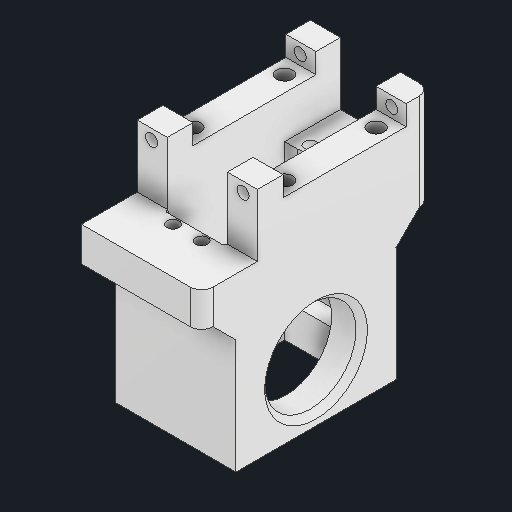
# Autodesk Inventor part: VerticalAxisServoMount
Saved by Autodesk Inventor 2025 (Build 290162000, 162)
## iProperties
Created: 2024-01-29
Part Number: VerticalAxisServoMount
Material: PC/ABS Plastic
Document SubType Name: Modeling
Designer: avsar
Density: 1.1 g/cm^3
Appearance: Smooth - White
Author: avsar
Autodesk Inventor part; units mm, degrees
ref_plane "YZ Plane" through (0, 0, 0) normal (1, 0, 0) x (0, 1, 0)
ref_plane "XZ Plane" through (0, 0, 0) normal (0, 1, 0) x (-1, 0, 0)
ref_plane "XY Plane" through (0, 0, 0) normal (0, 0, 1) x (1, 0, 0)
sketch "Sketch1" plane through (0, 0, 0) normal (1, 0, 0) x (0, 1, 0)
  circle A0 centre (0, 0) radius 15.95
  dimension "d0" = 31.9
  constraints: 1 centre point, 1 coincident
  measures "d0" diameter of A0
extrude "Extrusion1" add sketch "Sketch1" along normal blind 8
sketch "Sketch2" plane through (8, 0, 0) normal (1, 0, 0) x (0, 0, -1)
  line L0 (-28, -20) -> (28, -20)
  line L1 (28, -20) -> (28, 40)
  line L2 (28, 40) -> (-28, 40)
  line L3 (-28, 40) -> (-28, -20)
  line L4 (-28, -20) -> (28, 40) construction
  line L5 (28, -20) -> (-28, 40) construction
  point P0 (0, 0)
  point P1 (0, 10)
  point P2 (0, 10)
  dimension "d3" = 60
  dimension "d4" = 56
  dimension "d46" = 10
  constraints: 12 end point, 2 midpoint, 2 parallel, 1 horizontal, 1 perpendicular, 1 vertical alignment
  measures "d3" distance of L1.end L0.end
  measures "d4" distance of L1.end L2.end
  measures "d46" distance of point (0, 0) point (0, 10)
extrude "Extrusion2" add sketch "Sketch2" along normal blind 42
sketch "Sketch3" plane through (8, 40, 28) normal (0, 1, 0) x (1, 0, 0)
  line L0 (0, 56) -> (42, 56) projected
  line L1 (21, 56) -> (21, 0) construction
  line L2 (0, 0) -> (42, 0) projected
  line L3 (10.5, 7.5) -> (31.5, 7.5)
  line L4 (31.5, 7.5) -> (31.5, 48.5)
  line L5 (31.5, 48.5) -> (10.5, 48.5)
  line L6 (10.5, 48.5) -> (10.5, 7.5)
  line L7 (10.5, 7.5) -> (31.5, 48.5) construction
  line L8 (31.5, 7.5) -> (10.5, 48.5) construction
  point P0 (-8, 28)
  point P1 (21, 28)
  dimension "d7" = 21
  dimension "d8" = 41
  constraints: 14 end point, 5 midpoint, 2 parallel, 1 horizontal, 1 perpendicular
  measures "d7" distance of L5.end L4.end
  measures "d8" distance of L4.end L3.end
extrude "Extrusion3" cut sketch "Sketch3" against normal through all
sketch "Sketch4" plane through (50, 0, 0) normal (1, 0, 0) x (0, 0, -1)
  circle A0 centre (0, 0) radius 15.95 projected
extrude "Extrusion4" cut sketch "Sketch4" against normal up to surface (10.5 mm away)
sketch "Sketch5" plane through (18.5, 40, 20.5) normal (1, 0, 0) x (0, 0, -1)
  circle A0 centre (20.5, -40) radius 15.95 construction
  circle A1 centre (12.5, -32) radius 2.1
  circle A2 centre (12.5, -48) radius 2.1
  circle A3 centre (28.5, -48) radius 2.1
  circle A4 centre (28.5, -32) radius 2.1
  dimension "d13" = 4.2
  dimension "d14" = 8
  dimension "d15" = 8
  dimension "d18" = 360
  constraints: 4 centre point, 9 other
  measures "d13" diameter of A1
  measures "d14" horizontal distance of A1.centre point (20.5, -40)
  measures "d15" horizontal distance of point (20.5, -40) A1.centre
extrude "Extrusion5" cut sketch "Sketch5" against normal through all
sketch "Sketch6" plane through (8, 40, 28) normal (0, 1, 0) x (1, 0, 0)
  line L0 (31.5, 48.5) -> (10.5, 48.5) construction
  line L1 (21, 48.5) -> (21, 7.5) construction
  line L2 (10.5, 7.5) -> (31.5, 7.5) construction
  line L3 (0, 0) -> (42, 0) projected
  line L4 (0, 0) -> (42, 0)
  line L5 (42, 0) -> (42, -12)
  line L6 (42, -12) -> (0, -12)
  line L7 (0, -12) -> (0, 0)
  line L8 (10.5, 7.5) -> (10.5, 48.5) construction
  line L9 (10.5, 28) -> (31.5, 28) construction
  line L10 (31.5, 12.05) -> (31.5, 43.95) construction
  line L11 (0, 56) -> (42, 56)
  line L12 (0, 56) -> (42, 56)
  line L13 (42, 56) -> (42, 68)
  line L14 (42, 68) -> (0, 68)
  line L15 (0, 68) -> (0, 56)
  point P0 (-8, 28)
  point P1 (21, 28)
  dimension "d25" = 12
  constraints: 22 end point, 5 midpoint, 5 symmetric about line, 2 parallel, 1 coincident, 1 horizontal, 1 perpendicular
  measures "d25" distance of L4.end L5.end
extrude "Extrusion6" add sketch "Sketch6" against normal blind 12
sketch "Sketch8" plane through (8, 40, 40) normal (0, 1, 0) x (1, 0, 0)
  line L0 (10.5, 19.5) -> (31.5, 19.5) construction
  line L1 (21, 19.5) -> (21, 60.5) construction
  line L2 (31.5, 60.5) -> (10.5, 60.5) construction
  circle A0 centre (26, 16) radius 2.1
  line L3 (31.5, 19.5) -> (10.5, 19.5) projected
  line L4 (10.5, 19.5) -> (10.5, 60.5) construction
  line L5 (10.5, 40) -> (31.5, 40) construction
  line L6 (31.5, 24.05) -> (31.5, 55.95) construction
  circle A1 centre (16, 16) radius 2.1
  circle A2 centre (26, 64) radius 2.1
  circle A3 centre (16, 64) radius 2.1
  point P0 (-8, 40)
  point P1 (21, 40)
  dimension "d31" = 4.2
  dimension "d32" = 5
  dimension "d33" = 24
  constraints: 6 midpoint, 4 centre point, 4 end point, 3 symmetric about line, 3 other
  measures "d31" diameter of A0
  measures "d32" horizontal distance of point (21, 19.5) A0.centre
  measures "d33" vertical distance of point (21, 40) A0.centre
extrude "Extrusion8" cut sketch "Sketch8" against normal blind 8
fillet "Fillet2" radius 4 2 edges at (50, 34, 40) (50, 34, -40)
chamfer "Chamfer1" distance 2 angle 45 1 edges at (50, 0, 15.95)
chamfer "Chamfer2" distance 8 angle 45 2 edges at (29, 28, 28) (29, 28, -28)
sketch "Sketch10" plane through (8, 40, 40) normal (0, 1, 0) x (1, 0, 0)
  line L0 (31.5, 60.5) -> (10.5, 60.5) construction
  line L1 (21, 60.5) -> (21, 19.5) construction
  line L2 (31.5, 19.5) -> (10.5, 19.5) construction
  circle A0 centre (5, 33.97) radius 2.8
  circle A1 centre (5, 65.97) radius 2.8
  circle A2 centre (37, 33.97) radius 2.8
  circle A3 centre (37, 65.97) radius 2.8
  line L3 (0, 80) -> (0, 0) construction
  line L4 (0, 71.47) -> (10.5, 71.47)
  line L5 (10.5, 71.47) -> (10.5, 28.47)
  line L6 (10.5, 28.47) -> (0, 28.47)
  line L7 (0, 28.47) -> (0, 71.47)
  line L8 (5, 65.97) -> (5, 33.97) construction
  line L9 (42, 71.47) -> (31.5, 71.47)
  line L10 (31.5, 71.47) -> (31.5, 28.47)
  line L11 (31.5, 28.47) -> (42, 28.47)
  line L12 (42, 28.47) -> (42, 71.47)
  point P0 (-8, 40)
  point P1 (21, 40)
  point P2 (10.5, 49.97)
  point P3 (5, 49.97)
  dimension "d58" = 5.6
  dimension "d60" = 16
  dimension "d61" = 5.6
  dimension "d62" = 32
  dimension "d63" = 43
  dimension "d64" = 10.5
  dimension "d67" = 9.97
  constraints: 20 end point, 6 symmetric about line, 5 midpoint, 4 centre point, 2 parallel, 1 horizontal, 1 horizontal alignment, 1 perpendicular, 1 point on line, 1 vertical, 1 vertical alignment, 2 other
  measures "d58" diameter of A0
  measures "d60" horizontal distance of point (21, 40) L8.end
  measures "d61" diameter of A1
  measures "d62" distance of L8.end L8.start
  measures "d63" distance of L4.end L5.end
  measures "d64" distance of L4.start L4.end
  measures "d67" vertical distance of point (21, 40) point (5, 49.97)
extrude "Extrusion10" add sketch "Sketch10" along normal blind 14.8
sketch "Sketch11" plane through (0, 0, 0) normal (-1, 0, 0) x (0, 0, 1)
  circle A0 centre (-8, -8) radius 2.1 projected
  circle A1 centre (8, -8) radius 2.1 projected
  circle A2 centre (-8, 8) radius 2.1 projected
  circle A3 centre (8, 8) radius 2.1 projected
  circle A4 centre (0, 0) radius 15.95 projected
extrude "Extrusion11" cut sketch "Sketch11" against normal up to surface (8 mm away)
sketch "Sketch12" plane through (8, 0, 0) normal (-1, 0, 0) x (0, 0, 1)
  circle A0 centre (-8, 8) radius 2.1 projected
  circle A1 centre (-8, -8) radius 2.1 projected
  circle A2 centre (8, -8) radius 2.1 projected
  circle A3 centre (8, 8) radius 2.1 projected
  point P0 (0, 0)
sketch "Sketch13" plane through (8, 0, 0) normal (-1, 0, 0) x (0, 0, 1)
  circle A0 centre (0, 11) radius 1.3
  circle A1 centre (-7.7782, 7.7782) radius 1.3
  circle A2 centre (-11, 0) radius 1.3
  circle A3 centre (-7.7782, -7.7782) radius 1.3
  circle A4 centre (0, -11) radius 1.3
  circle A5 centre (7.7782, -7.7782) radius 1.3
  circle A6 centre (11, 0) radius 1.3
  circle A7 centre (7.7782, 7.7782) radius 1.3
  point P0 (0, 0)
  dimension "d70" = 2.6
  dimension "d71" = 11
  dimension "d76" = 360
  constraints: 8 centre point, 1 vertical alignment, 17 other
  measures "d70" diameter of A0
  measures "d71" distance of point (0, 0) A0.centre
extrude "Extrusion12" add sketch "Sketch12" against normal up to surface (10.5 mm away)
extrude "Extrusion13" cut sketch "Sketch13" against normal through all
sketch "Sketch14" plane through (18.5, 40, 20.5) normal (0, 1, 0) x (1, 0, 0)
  line L0 (-10.5, 8.97) -> (-10.5, -19.5) projected
  line L1 (0, 41) -> (0, 0) projected
  line L2 (-10.5, 8.97) -> (0, 8.97)
  line L3 (0, 8.97) -> (0, 0)
  line L4 (0, 0) -> (-10.5, 0)
  line L5 (-10.5, 0) -> (-10.5, 8.97)
  line L6 (31.5, 8.97) -> (21, 8.97) projected
  line L7 (31.5, -7.5) -> (31.5, 48.5) projected
  line L8 (21, 8.97) -> (31.5, 8.97)
  line L9 (31.5, 8.97) -> (31.5, 0)
  line L10 (31.5, 0) -> (21, 0)
  line L11 (21, 0) -> (21, 8.97)
  line L12 (-10.5, 51.97) -> (0, 51.97) projected
  line L13 (-10.5, 60.5) -> (27.5, 60.5) projected
  line L14 (-10.5, 51.97) -> (0, 51.97)
  line L15 (0, 51.97) -> (0, 60.5)
  line L16 (0, 60.5) -> (-10.5, 60.5)
  line L17 (-10.5, 60.5) -> (-10.5, 51.97)
  line L18 (31.5, 51.97) -> (21, 51.97)
  line L19 (21, 51.97) -> (21, 60.5)
  line L20 (21, 60.5) -> (27.5, 60.5)
  line L21 (31.5, 56.5) -> (31.5, 51.97)
  arc A0 (31.5, 56.5) -> (27.5, 60.5) centre (27.5, 56.5) ccw
  point P0 (-18.5, 20.5)
  point P1 (0, 8.97)
  point P2 (27.5, 60.5)
  dimension "d82" = 4
  constraints: 32 end point, 8 parallel, 4 horizontal, 4 perpendicular, 4 point on line, 2 point on circle, 2 tangent, 1 centre point, 1 horizontal alignment
  measures "d82" radius of A0
extrude "Extrusion14" add sketch "Sketch14" along normal blind 21.8
sketch "Sketch15" plane through (8, 40, 20.5) normal (0, 0, 1) x (1, 0, 0)
  circle A0 centre (5, 18.3) radius 2.1
  line L0 (10.5, 14.8) -> (0, 14.8) construction
  line L1 (10.5, 14.8) -> (10.5, 21.8) construction
  line L2 (0, 21.8) -> (10.5, 21.8) construction
  line L3 (0, 14.8) -> (0, 21.8) construction
  line L4 (31.5, 0) -> (10.5, 0) projected
  line L5 (21, 0) -> (21, 26.153) construction
  circle A1 centre (37, 18.3) radius 2.1
  point P0 (-8, -40)
  point P1 (5.25, 14.8)
  dimension "d83" = 4.2
  dimension "d84" = 3.5
  dimension "d87" = 0.25
  constraints: 2 centre point, 2 end point, 2 midpoint, 1 symmetric about line, 1 vertical, 1 other
  measures "d83" diameter of A0
  measures "d84" vertical distance of point (5.25, 14.8) A0.centre
  measures "d87" horizontal distance of point (5.25, 14.8) A0.centre
extrude "Extrusion15" cut sketch "Sketch15" against normal through all
sketch "Sketch16" plane through (8, -20, -28) normal (0, -1, 0) x (1, 0, 0)
  line L0 (13, 13.5) -> (29, 13.5)
  line L1 (29, 13.5) -> (29, 1.5)
  line L2 (29, 1.5) -> (13, 1.5)
  line L3 (13, 1.5) -> (13, 13.5)
  line L4 (31.5, 7.5) -> (10.5, 7.5) projected
  line L5 (13, 13.5) -> (29, 1.5) construction
  line L6 (29, 13.5) -> (13, 1.5) construction
  point P0 (-8, 28)
  point P1 (21, 7.5)
  point P2 (29, 7.5)
  point P3 (13, 7.5)
  dimension "d88" = 16
  dimension "d89" = 12
  constraints: 12 end point, 3 midpoint, 2 parallel, 1 horizontal, 1 perpendicular
  measures "d88" distance of L1.end L2.end
  measures "d89" distance of L0.end L1.end
extrude "Extrusion16" cut sketch "Sketch16" against normal blind 52 contours L4 L1 L2 L3
extrude "Extrusion17" add sketch "Sketch16" against normal blind 12 contours L4 L1 L2 L3
sketch "Sketch17" plane through (18.5, 40, -20.5) normal (0, 1, 0) x (1, 0, 0)
  line L0 (0, 0) -> (21, 0) projected
  line L1 (8.5, 0) -> (12.5, 0)
  line L2 (12.5, 0) -> (12.5, 6)
  line L3 (12.5, 6) -> (8.5, 6)
  line L4 (8.5, 6) -> (8.5, 0)
  point P0 (-18.5, -20.5)
  point P1 (10.5, 0)
  point P2 (12.5, 0)
  dimension "d94" = 4
  dimension "d95" = 6
  constraints: 8 end point, 2 midpoint, 2 parallel, 1 horizontal, 1 perpendicular, 1 point on line
  measures "d94" distance of L2.end L3.end
  measures "d95" distance of L1.end L2.end
extrude "Extrusion18" cut sketch "Sketch17" against normal blind 13.8125
fillet "Fillet3" radius 2 2 edges at (27, 36, -26.5) (31, 36, -26.5)
fillet "Fillet4" radius 4 2 edges at (27, 36, -20.5) (31, 36, -20.5)
chamfer "Chamfer3" distance 1 angle 45 1 edges at (29, 40, 20.5)
chamfer "Chamfer4" distance 0.7 angle 45 2 edges at (18.5, 39.5, 21) (39.5, 39.5, 21)
body "Solid1"
